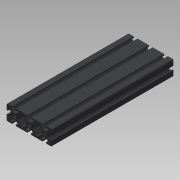
# Autodesk Inventor part: 1545-S
Saved by Autodesk Inventor 2013 (Build 170138000, 138)
## iProperties
Company: 80/20 Inc.
Created: 2014-04-23
Part Number: 1545-S
Material: Generic
Document SubType Name: Modeling
Density: 1 g/cm^3
Vendor: 80/20 Inc.
Engineer: Ross Bowman
Designer: Ross Bowman
Catalog Web Link: 8020.net
Material: 6105-T5 Aluminum
Author: Ross Bowman
Keywords: 80/20 , 8020 , T-Slot , Extrusion
Autodesk Inventor part; units mm, degrees
ref_plane "YZ Plane" through (0, 0, 0) normal (1, 0, 0) x (0, 1, 0)
ref_plane "XZ Plane" through (0, 0, 0) normal (0, 1, 0) x (-1, 0, 0)
ref_plane "XY Plane" through (0, 0, 0) normal (0, 0, 1) x (1, 0, 0)
sketch "Sketch1" plane through (0, 0, 0) normal (0, 0, 1) x (1, 0, 0)
  arc A0 (-21.1155, -14.1109) -> (-16.9845, -14.1109) centre (-19.05, -12.0454) ccw
  line L0 (-29.8392, -5.3872) -> (-21.1155, -14.1109)
  arc A1 (-31.2303, -2.0285) -> (-29.8392, -5.3872) centre (-26.4805, -2.0285) ccw
  line L1 (-31.2303, 2.0285) -> (-31.2303, -2.0285)
  arc A2 (-29.8392, 5.3872) -> (-31.2303, 2.0285) centre (-26.4805, 2.0285) ccw
  line L2 (-21.1155, 14.1109) -> (-29.8392, 5.3872)
  arc A3 (-16.9845, 14.1109) -> (-21.1155, 14.1109) centre (-19.05, 12.0454) ccw
  line L3 (-8.2608, 5.3872) -> (-16.9845, 14.1109)
  arc A4 (-6.8697, 2.0285) -> (-8.2608, 5.3872) centre (-11.6195, 2.0285) ccw
  line L4 (-6.8697, -2.0285) -> (-6.8697, 2.0285)
  arc A5 (-8.2608, -5.3872) -> (-6.8697, -2.0285) centre (-11.6195, -2.0285) ccw
  line L5 (-16.9845, -14.1109) -> (-8.2608, -5.3872)
  arc A6 (-35.3731, -4.3433) -> (-33.7567, -2.7269) centre (-34.5649, -3.5351) ccw
  line L6 (-36.7436, -2.9729) -> (-35.3731, -4.3433)
  arc A7 (-39.4564, -2.9729) -> (-36.7436, -2.9729) centre (-38.1, 0) ccw
  line L7 (-40.8269, -4.3433) -> (-39.4564, -2.9729)
  arc A8 (-42.4433, -2.7269) -> (-40.8269, -4.3433) centre (-41.6351, -3.5351) ccw
  line L8 (-41.0729, -1.3564) -> (-42.4433, -2.7269)
  arc A9 (-41.0729, 1.3564) -> (-41.0729, -1.3564) centre (-38.1, 0) ccw
  line L9 (-42.3456, 2.6398) -> (-41.0729, 1.3564)
  arc A10 (-40.7398, 4.2456) -> (-42.3456, 2.6398) centre (-41.6351, 3.5351) ccw
  line L10 (-39.4564, 2.9729) -> (-40.7398, 4.2456)
  arc A11 (-36.7436, 2.9729) -> (-39.4564, 2.9729) centre (-38.1, 0) ccw
  line L11 (-35.3731, 4.3433) -> (-36.7436, 2.9729)
  arc A12 (-33.7567, 2.7269) -> (-35.3731, 4.3433) centre (-34.5649, 3.5351) ccw
  line L12 (-35.1271, 1.3564) -> (-33.7567, 2.7269)
  arc A13 (-35.1271, -1.3564) -> (-35.1271, 1.3564) centre (-38.1, 0) ccw
  line L13 (-33.7567, -2.7269) -> (-35.1271, -1.3564)
  arc A14 (33.7567, -2.7269) -> (35.3731, -4.3433) centre (34.5649, -3.5351) ccw
  line L14 (35.1271, -1.3564) -> (33.7567, -2.7269)
  arc A15 (35.1271, 1.3564) -> (35.1271, -1.3564) centre (38.1, 0) ccw
  line L15 (33.7567, 2.7269) -> (35.1271, 1.3564)
  arc A16 (35.3731, 4.3433) -> (33.7567, 2.7269) centre (34.5649, 3.5351) ccw
  line L16 (36.7436, 2.9729) -> (35.3731, 4.3433)
  arc A17 (39.4564, 2.9729) -> (36.7436, 2.9729) centre (38.1, 0) ccw
  line L17 (40.7398, 4.2456) -> (39.4564, 2.9729)
  arc A18 (42.3456, 2.6398) -> (40.7398, 4.2456) centre (41.6351, 3.5351) ccw
  line L18 (41.0729, 1.3564) -> (42.3456, 2.6398)
  arc A19 (41.0729, -1.3564) -> (41.0729, 1.3564) centre (38.1, 0) ccw
  line L19 (42.4433, -2.7269) -> (41.0729, -1.3564)
  arc A20 (40.8269, -4.3433) -> (42.4433, -2.7269) centre (41.6351, -3.5351) ccw
  line L20 (39.4564, -2.9729) -> (40.8269, -4.3433)
  arc A21 (36.7436, -2.9729) -> (39.4564, -2.9729) centre (38.1, 0) ccw
  line L21 (35.3731, -4.3433) -> (36.7436, -2.9729)
  arc A22 (16.9845, -14.1109) -> (21.1155, -14.1109) centre (19.05, -12.0454) ccw
  line L22 (8.2608, -5.3872) -> (16.9845, -14.1109)
  arc A23 (6.8697, -2.0285) -> (8.2608, -5.3872) centre (11.6195, -2.0285) ccw
  line L23 (6.8697, 2.0285) -> (6.8697, -2.0285)
  arc A24 (8.2608, 5.3872) -> (6.8697, 2.0285) centre (11.6195, 2.0285) ccw
  line L24 (16.9845, 14.1109) -> (8.2608, 5.3872)
  arc A25 (21.1155, 14.1109) -> (16.9845, 14.1109) centre (19.05, 12.0454) ccw
  line L25 (29.8392, 5.3872) -> (21.1155, 14.1109)
  arc A26 (31.2303, 2.0285) -> (29.8392, 5.3872) centre (26.4805, 2.0285) ccw
  line L26 (31.2303, -2.0285) -> (31.2303, 2.0285)
  arc A27 (29.8392, -5.3872) -> (31.2303, -2.0285) centre (26.4805, -2.0285) ccw
  line L27 (21.1155, -14.1109) -> (29.8392, -5.3872)
  arc A28 (-4.3433, -2.7269) -> (-2.7269, -4.3433) centre (-3.5351, -3.5351) ccw
  line L28 (-2.9729, -1.3564) -> (-4.3433, -2.7269)
  arc A29 (-2.9729, 1.3564) -> (-2.9729, -1.3564) centre (0, 0) ccw
  line L29 (-4.3433, 2.7269) -> (-2.9729, 1.3564)
  arc A30 (-2.7269, 4.3433) -> (-4.3433, 2.7269) centre (-3.5351, 3.5351) ccw
  line L30 (-1.3564, 2.9729) -> (-2.7269, 4.3433)
  arc A31 (1.3564, 2.9729) -> (-1.3564, 2.9729) centre (0, 0) ccw
  line L31 (2.7269, 4.3433) -> (1.3564, 2.9729)
  arc A32 (4.3433, 2.7269) -> (2.7269, 4.3433) centre (3.5351, 3.5351) ccw
  line L32 (2.9729, 1.3564) -> (4.3433, 2.7269)
  arc A33 (2.9729, -1.3564) -> (2.9729, 1.3564) centre (0, 0) ccw
  line L33 (4.3433, -2.7269) -> (2.9729, -1.3564)
  arc A34 (2.7269, -4.3433) -> (4.3433, -2.7269) centre (3.5351, -3.5351) ccw
  line L34 (1.3564, -2.9729) -> (2.7269, -4.3433)
  arc A35 (-1.3564, -2.9729) -> (1.3564, -2.9729) centre (0, 0) ccw
  line L35 (-2.7269, -4.3433) -> (-1.3564, -2.9729)
  arc A36 (-42.164, -16.5608) -> (-43.7388, -14.986) centre (-43.7388, -16.5608) ccw
  line L36 (-43.7388, -14.986) -> (-47.498, -14.986)
  arc A37 (-48.387, -14.097) -> (-47.498, -14.986) centre (-47.498, -14.097) ccw
  line L37 (-48.387, -14.097) -> (-48.387, -13.5289)
  arc A38 (-48.1266, -12.9003) -> (-48.387, -13.5289) centre (-47.498, -13.5289) ccw
  line L38 (-48.1266, -12.9003) -> (-43.4872, -8.2608)
  arc A39 (-40.1285, -6.8697) -> (-43.4872, -8.2608) centre (-40.1285, -11.6195) ccw
  line L39 (-40.1285, -6.8697) -> (-36.0715, -6.8697)
  arc A40 (-32.7128, -8.2608) -> (-36.0715, -6.8697) centre (-36.0715, -11.6195) ccw
  line L40 (-32.7128, -8.2608) -> (-28.0734, -12.9003)
  arc A41 (-27.813, -13.5289) -> (-28.0734, -12.9003) centre (-28.702, -13.5289) ccw
  line L41 (-27.813, -13.5289) -> (-27.813, -14.097)
  arc A42 (-28.702, -14.986) -> (-27.813, -14.097) centre (-28.702, -14.097) ccw
  line L42 (-28.702, -14.986) -> (-32.4612, -14.986)
  arc A43 (-32.4612, -14.986) -> (-34.036, -16.5608) centre (-32.4612, -16.5608) ccw
  line L43 (-34.036, -16.5608) -> (-34.036, -17.4752)
  arc A44 (-34.036, -17.4752) -> (-32.4612, -19.05) centre (-32.4612, -17.4752) ccw
  line L44 (-32.4612, -19.05) -> (-5.6388, -19.05)
  arc A45 (-5.6388, -19.05) -> (-4.064, -17.4752) centre (-5.6388, -17.4752) ccw
  line L45 (-4.064, -17.4752) -> (-4.064, -16.5608)
  arc A46 (-4.064, -16.5608) -> (-5.6388, -14.986) centre (-5.6388, -16.5608) ccw
  line L46 (-5.6388, -14.986) -> (-9.398, -14.986)
  arc A47 (-10.287, -14.097) -> (-9.398, -14.986) centre (-9.398, -14.097) ccw
  line L47 (-10.287, -14.097) -> (-10.287, -13.5289)
  arc A48 (-10.0266, -12.9003) -> (-10.287, -13.5289) centre (-9.398, -13.5289) ccw
  line L48 (-10.0266, -12.9003) -> (-5.3872, -8.2608)
  arc A49 (-2.0285, -6.8697) -> (-5.3872, -8.2608) centre (-2.0285, -11.6195) ccw
  line L49 (-2.0285, -6.8697) -> (2.0285, -6.8697)
  arc A50 (5.3872, -8.2608) -> (2.0285, -6.8697) centre (2.0285, -11.6195) ccw
  line L50 (5.3872, -8.2608) -> (10.0266, -12.9003)
  arc A51 (10.287, -13.5289) -> (10.0266, -12.9003) centre (9.398, -13.5289) ccw
  line L51 (10.287, -13.5289) -> (10.287, -14.097)
  arc A52 (9.398, -14.986) -> (10.287, -14.097) centre (9.398, -14.097) ccw
  line L52 (9.398, -14.986) -> (5.6388, -14.986)
  arc A53 (5.6388, -14.986) -> (4.064, -16.5608) centre (5.6388, -16.5608) ccw
  line L53 (4.064, -16.5608) -> (4.064, -17.4752)
  arc A54 (4.064, -17.4752) -> (5.6388, -19.05) centre (5.6388, -17.4752) ccw
  line L54 (5.6388, -19.05) -> (32.4612, -19.05)
  arc A55 (32.4612, -19.05) -> (34.036, -17.4752) centre (32.4612, -17.4752) ccw
  line L55 (34.036, -17.4752) -> (34.036, -16.5608)
  arc A56 (34.036, -16.5608) -> (32.4612, -14.986) centre (32.4612, -16.5608) ccw
  line L56 (32.4612, -14.986) -> (28.702, -14.986)
  arc A57 (27.813, -14.097) -> (28.702, -14.986) centre (28.702, -14.097) ccw
  line L57 (27.813, -14.097) -> (27.813, -13.5289)
  arc A58 (28.0734, -12.9003) -> (27.813, -13.5289) centre (28.702, -13.5289) ccw
  line L58 (28.0734, -12.9003) -> (32.7128, -8.2608)
  arc A59 (36.0715, -6.8697) -> (32.7128, -8.2608) centre (36.0715, -11.6195) ccw
  line L59 (36.0715, -6.8697) -> (40.1285, -6.8697)
  arc A60 (43.4872, -8.2608) -> (40.1285, -6.8697) centre (40.1285, -11.6195) ccw
  line L60 (43.4872, -8.2608) -> (48.1266, -12.9003)
  arc A61 (48.387, -13.5289) -> (48.1266, -12.9003) centre (47.498, -13.5289) ccw
  line L61 (48.387, -13.5289) -> (48.387, -14.097)
  arc A62 (47.498, -14.986) -> (48.387, -14.097) centre (47.498, -14.097) ccw
  line L62 (47.498, -14.986) -> (43.7388, -14.986)
  arc A63 (43.7388, -14.986) -> (42.164, -16.5608) centre (43.7388, -16.5608) ccw
  line L63 (42.164, -16.5608) -> (42.164, -17.4752)
  arc A64 (42.164, -17.4752) -> (43.7388, -19.05) centre (43.7388, -17.4752) ccw
  line L64 (43.7388, -19.05) -> (53.975, -19.05)
  arc A65 (53.975, -19.05) -> (57.15, -15.875) centre (53.975, -15.875) ccw
  line L65 (57.15, -15.875) -> (57.15, -5.6388)
  arc A66 (57.15, -5.6388) -> (55.5752, -4.064) centre (55.5752, -5.6388) ccw
  line L66 (55.5752, -4.064) -> (54.6608, -4.064)
  arc A67 (54.6608, -4.064) -> (53.086, -5.6388) centre (54.6608, -5.6388) ccw
  line L67 (53.086, -5.6388) -> (53.086, -9.398)
  arc A68 (52.197, -10.287) -> (53.086, -9.398) centre (52.197, -9.398) ccw
  line L68 (52.197, -10.287) -> (51.6289, -10.287)
  arc A69 (51.0003, -10.0266) -> (51.6289, -10.287) centre (51.6289, -9.398) ccw
  line L69 (51.0003, -10.0266) -> (46.3608, -5.3872)
  arc A70 (44.9697, -2.0285) -> (46.3608, -5.3872) centre (49.7195, -2.0285) ccw
  line L70 (44.9697, -2.0285) -> (44.9697, 2.0285)
  arc A71 (46.3608, 5.3872) -> (44.9697, 2.0285) centre (49.7195, 2.0285) ccw
  line L71 (46.3608, 5.3872) -> (51.0003, 10.0266)
  arc A72 (51.6289, 10.287) -> (51.0003, 10.0266) centre (51.6289, 9.398) ccw
  line L72 (51.6289, 10.287) -> (52.197, 10.287)
  arc A73 (53.086, 9.398) -> (52.197, 10.287) centre (52.197, 9.398) ccw
  line L73 (53.086, 9.398) -> (53.086, 5.6388)
  arc A74 (53.086, 5.6388) -> (54.6608, 4.064) centre (54.6608, 5.6388) ccw
  line L74 (54.6608, 4.064) -> (55.5752, 4.064)
  arc A75 (55.5752, 4.064) -> (57.15, 5.6388) centre (55.5752, 5.6388) ccw
  line L75 (57.15, 5.6388) -> (57.15, 15.875)
  arc A76 (57.15, 15.875) -> (53.975, 19.05) centre (53.975, 15.875) ccw
  line L76 (53.975, 19.05) -> (43.7388, 19.05)
  arc A77 (43.7388, 19.05) -> (42.164, 17.4752) centre (43.7388, 17.4752) ccw
  line L77 (42.164, 17.4752) -> (42.164, 16.5608)
  arc A78 (42.164, 16.5608) -> (43.7388, 14.986) centre (43.7388, 16.5608) ccw
  line L78 (43.7388, 14.986) -> (47.498, 14.986)
  arc A79 (48.387, 14.097) -> (47.498, 14.986) centre (47.498, 14.097) ccw
  line L79 (48.387, 14.097) -> (48.387, 13.5289)
  arc A80 (48.1266, 12.9003) -> (48.387, 13.5289) centre (47.498, 13.5289) ccw
  line L80 (48.1266, 12.9003) -> (43.4872, 8.2608)
  arc A81 (40.1285, 6.8697) -> (43.4872, 8.2608) centre (40.1285, 11.6195) ccw
  line L81 (40.1285, 6.8697) -> (36.0715, 6.8697)
  arc A82 (32.7128, 8.2608) -> (36.0715, 6.8697) centre (36.0715, 11.6195) ccw
  line L82 (32.7128, 8.2608) -> (28.0734, 12.9003)
  arc A83 (27.813, 13.5289) -> (28.0734, 12.9003) centre (28.702, 13.5289) ccw
  line L83 (27.813, 13.5289) -> (27.813, 14.097)
  arc A84 (28.702, 14.986) -> (27.813, 14.097) centre (28.702, 14.097) ccw
  line L84 (28.702, 14.986) -> (32.4612, 14.986)
  arc A85 (32.4612, 14.986) -> (34.036, 16.5608) centre (32.4612, 16.5608) ccw
  line L85 (34.036, 16.5608) -> (34.036, 17.4752)
  arc A86 (34.036, 17.4752) -> (32.4612, 19.05) centre (32.4612, 17.4752) ccw
  line L86 (32.4612, 19.05) -> (5.6388, 19.05)
  arc A87 (5.6388, 19.05) -> (4.064, 17.4752) centre (5.6388, 17.4752) ccw
  line L87 (4.064, 17.4752) -> (4.064, 16.5608)
  arc A88 (4.064, 16.5608) -> (5.6388, 14.986) centre (5.6388, 16.5608) ccw
  line L88 (5.6388, 14.986) -> (9.398, 14.986)
  arc A89 (10.287, 14.097) -> (9.398, 14.986) centre (9.398, 14.097) ccw
  line L89 (10.287, 14.097) -> (10.287, 13.5289)
  arc A90 (10.0266, 12.9003) -> (10.287, 13.5289) centre (9.398, 13.5289) ccw
  line L90 (10.0266, 12.9003) -> (5.3872, 8.2608)
  arc A91 (2.0285, 6.8697) -> (5.3872, 8.2608) centre (2.0285, 11.6195) ccw
  line L91 (2.0285, 6.8697) -> (-2.0285, 6.8697)
  arc A92 (-5.3872, 8.2608) -> (-2.0285, 6.8697) centre (-2.0285, 11.6195) ccw
  line L92 (-5.3872, 8.2608) -> (-10.0266, 12.9003)
  arc A93 (-10.287, 13.5289) -> (-10.0266, 12.9003) centre (-9.398, 13.5289) ccw
  line L93 (-10.287, 13.5289) -> (-10.287, 14.097)
  arc A94 (-9.398, 14.986) -> (-10.287, 14.097) centre (-9.398, 14.097) ccw
  line L94 (-9.398, 14.986) -> (-5.6388, 14.986)
  arc A95 (-5.6388, 14.986) -> (-4.064, 16.5608) centre (-5.6388, 16.5608) ccw
  line L95 (-4.064, 16.5608) -> (-4.064, 17.4752)
  arc A96 (-4.064, 17.4752) -> (-5.6388, 19.05) centre (-5.6388, 17.4752) ccw
  line L96 (-5.6388, 19.05) -> (-32.4612, 19.05)
  arc A97 (-32.4612, 19.05) -> (-34.036, 17.4752) centre (-32.4612, 17.4752) ccw
  line L97 (-34.036, 17.4752) -> (-34.036, 16.5608)
  arc A98 (-34.036, 16.5608) -> (-32.4612, 14.986) centre (-32.4612, 16.5608) ccw
  line L98 (-32.4612, 14.986) -> (-28.702, 14.986)
  arc A99 (-27.813, 14.097) -> (-28.702, 14.986) centre (-28.702, 14.097) ccw
  line L99 (-27.813, 14.097) -> (-27.813, 13.5289)
  arc A100 (-28.0734, 12.9003) -> (-27.813, 13.5289) centre (-28.702, 13.5289) ccw
  line L100 (-28.0734, 12.9003) -> (-32.7128, 8.2608)
  arc A101 (-36.0715, 6.8697) -> (-32.7128, 8.2608) centre (-36.0715, 11.6195) ccw
  line L101 (-36.0715, 6.8697) -> (-40.1285, 6.8697)
  arc A102 (-43.4872, 8.2608) -> (-40.1285, 6.8697) centre (-40.1285, 11.6195) ccw
  line L102 (-43.4872, 8.2608) -> (-48.1266, 12.9003)
  arc A103 (-48.387, 13.5289) -> (-48.1266, 12.9003) centre (-47.498, 13.5289) ccw
  line L103 (-48.387, 13.5289) -> (-48.387, 14.097)
  arc A104 (-47.498, 14.986) -> (-48.387, 14.097) centre (-47.498, 14.097) ccw
  line L104 (-47.498, 14.986) -> (-43.7388, 14.986)
  arc A105 (-43.7388, 14.986) -> (-42.164, 16.5608) centre (-43.7388, 16.5608) ccw
  line L105 (-42.164, 16.5608) -> (-42.164, 17.4752)
  arc A106 (-42.164, 17.4752) -> (-43.7388, 19.05) centre (-43.7388, 17.4752) ccw
  line L106 (-43.7388, 19.05) -> (-53.975, 19.05)
  arc A107 (-53.975, 19.05) -> (-57.15, 15.875) centre (-53.975, 15.875) ccw
  line L107 (-57.15, 15.875) -> (-57.15, 5.6388)
  arc A108 (-57.15, 5.6388) -> (-55.5752, 4.064) centre (-55.5752, 5.6388) ccw
  line L108 (-55.5752, 4.064) -> (-54.6608, 4.064)
  arc A109 (-54.6608, 4.064) -> (-53.086, 5.6388) centre (-54.6608, 5.6388) ccw
  line L109 (-53.086, 5.6388) -> (-53.086, 9.398)
  arc A110 (-52.197, 10.287) -> (-53.086, 9.398) centre (-52.197, 9.398) ccw
  line L110 (-52.197, 10.287) -> (-51.6289, 10.287)
  arc A111 (-51.0003, 10.0266) -> (-51.6289, 10.287) centre (-51.6289, 9.398) ccw
  line L111 (-51.0003, 10.0266) -> (-46.3608, 5.3872)
  arc A112 (-44.9697, 2.0285) -> (-46.3608, 5.3872) centre (-49.7195, 2.0285) ccw
  line L112 (-44.9697, 2.0285) -> (-44.9697, -2.0285)
  arc A113 (-46.3608, -5.3872) -> (-44.9697, -2.0285) centre (-49.7195, -2.0285) ccw
  line L113 (-46.3608, -5.3872) -> (-51.0003, -10.0266)
  arc A114 (-51.6289, -10.287) -> (-51.0003, -10.0266) centre (-51.6289, -9.398) ccw
  line L114 (-51.6289, -10.287) -> (-52.197, -10.287)
  arc A115 (-53.086, -9.398) -> (-52.197, -10.287) centre (-52.197, -9.398) ccw
  line L115 (-53.086, -9.398) -> (-53.086, -5.6388)
  arc A116 (-53.086, -5.6388) -> (-54.6608, -4.064) centre (-54.6608, -5.6388) ccw
  line L116 (-54.6608, -4.064) -> (-55.5752, -4.064)
  arc A117 (-55.5752, -4.064) -> (-57.15, -5.6388) centre (-55.5752, -5.6388) ccw
  line L117 (-57.15, -5.6388) -> (-57.15, -15.875)
  arc A118 (-57.15, -15.875) -> (-53.975, -19.05) centre (-53.975, -15.875) ccw
  line L118 (-53.975, -19.05) -> (-43.7388, -19.05)
  arc A119 (-43.7388, -19.05) -> (-42.164, -17.4752) centre (-43.7388, -17.4752) ccw
  line L119 (-42.164, -17.4752) -> (-42.164, -16.5608)
  constraints: 240 end point, 240 point on circle, 120 centre point
extrude "Extrusion1" add sketch "Sketch1" against normal blind 304.8
body "Solid1"
